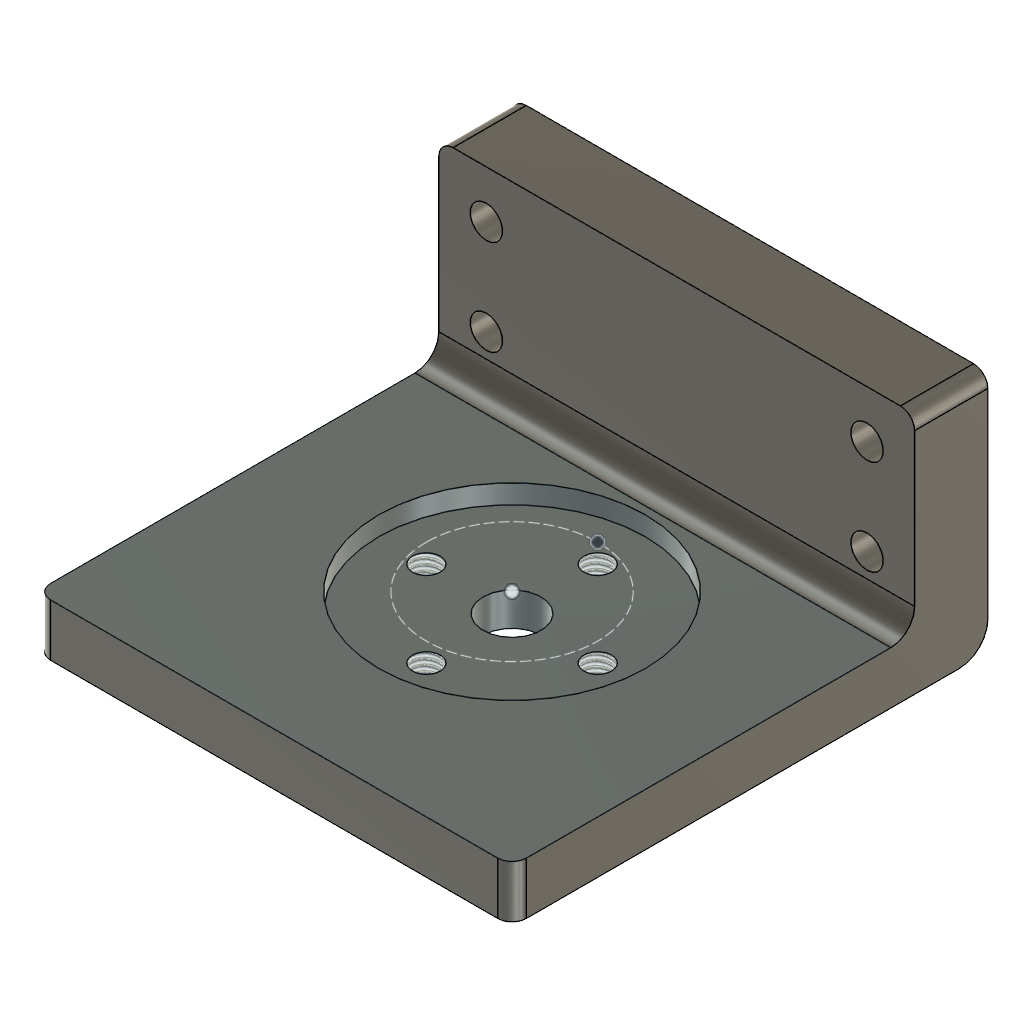
Motor Mount (Autodesk Fusion 360 design; units mm, degrees)
part number: 2026-09-16-15-06-11-104
Autodesk Fusion 360 part; units mm, degrees
sketch "Sketch1" plane through (0, 0, 0) normal (0, 0, 1) x (1, 0, 0)
  line L0 (25, 25) -> (-25, 25)
  line L1 (-25, 25) -> (-25, -25)
  line L2 (-25, -25) -> (25, -25)
  line L3 (25, -25) -> (25, 25)
  line L4 (25, 25) -> (-25, -25) construction
  line L5 (-25, 25) -> (25, -25) construction
  dimension "d1" = 50
  dimension "d2" = 50
  constraint horizontal L0
  constraint perpendicular L0 L1
  constraint parallel L0 L2
  constraint parallel L1 L3
  constraint coincident L4 origin
  constraint coincident L5 origin
  measures "d1" distance of L0.end L1.end
  measures "d2" distance of L0.start L0.end
extrude "Extrude1" add sketch "Sketch1" along normal blind 5.5
sketch "Sketch2" plane through (0, 0, 5.5) normal (0, 0, 1) x (-1, 0, 0)
  line L0 (-25, 25) -> (-25, -25)
  line L1 (-25, -25) -> (25, -25)
  line L2 (25, -25) -> (25, 25)
  line L3 (25, 25) -> (-25, 25)
  line L4 (25, -25) -> (-25, -25)
  line L5 (-25, -25) -> (-25, -17.3)
  line L6 (-25, -17.3) -> (25, -17.3)
  line L7 (25, -17.3) -> (25, -25)
  dimension "d11" = 7.7
  dimension "d12" = 50
  constraint horizontal L4
  constraint vertical L5
  constraint horizontal L6
  constraint vertical L7
  constraint coincident L1.end L2.start
  measures "d11" distance of L1.end L6.end
  measures "d12" distance of L1.end L0.end
extrude "Extrude2" add sketch "Sketch2" along normal blind 20 contours L0 L1 L2 L4 L5 L6 L7
sketch "Sketch3" plane through (0, 0, 5.5) normal (0, 0, 1) x (-1, 0, 0)
  line L0 (-25, -17.3) -> (25, -17.3)
  line L1 (25, -17.3) -> (25, 25)
  line L2 (25, 25) -> (-25, 25)
  line L3 (-25, 25) -> (-25, -17.3)
  circle A0 centre (0, 0) radius 14
  dimension "d15" = 28
  constraint coincident A0.centre origin
  measures "d15" diameter of A0
sketch "Sketch4" plane through (0, 0, 5.5) normal (0, 0, 1) x (-1, 0, 0)
fillet "Fillet1" radius 2.5 1 edges at (0, 17.3, 5.5)
fillet "Fillet2" radius 3 1 edges at (0, 25, 0)
fillet "Fillet3" radius 1.5 4 edges at (25, -25, 2.75) (-25, -25, 2.75) (25, 21.15, 25.5) (-25, 21.15, 25.5)
extrude "Extrude3" cut sketch "Sketch3" against normal blind 2 contours A0
sketch "Sketch5" plane through (0, 0, 5.5) normal (0, 0, 1) x (-1, 0, 0)
  circle A0 centre (0, 0) radius 14
  arc A1 (25, 23.5) -> (23.5, 25) centre (23.5, 23.5) ccw
  line L0 (23.5, 25) -> (-23.5, 25)
  arc A2 (-23.5, 25) -> (-25, 23.5) centre (-23.5, 23.5) ccw
  line L1 (-25, 23.5) -> (-25, -14.8)
  line L2 (-25, -14.8) -> (25, -14.8)
  line L3 (25, -14.8) -> (25, 23.5)
  circle A3 centre (0, 0) radius 9 construction
  point P0 (0, -9)
  dimension "d24" = 18
  constraint concentric A0 A3
  constraint coincident A3 P0
  measures "d24" diameter of A3
hole "Hole1" at (0, 0, 5.5) direction (0, 0, -1) diameter 6.1 depth 10 tip angle 118
hole "Hole2" at (0, 9, 5.5) direction (0, 0, -1) diameter 2.93 depth 10 tip angle 118
thread "Thread1" "ISO Metric profile 3.5 M3.5x0.6 M3.5x0.6 6H" thread offset 0 thread depth 7.4
pattern_circular "C-Pattern1" count 4 over 360 about axis through (0, 0, 1.75) along (0, 0, 1) of "Hole2"
hole "Hole3" at (-20, 17.3, 20.5) direction (0, 1, 0) diameter 3.4 depth 10 tip angle 118
hole "Hole4" at (-20, 17.3, 10.5) direction (0, 1, 0) diameter 3.4 depth 10 tip angle 118
hole "Hole5" at (20, 17.3, 20.5) direction (0, 1, 0) diameter 3.4 depth 10 tip angle 118
hole "Hole6" at (20, 17.3, 10.5) direction (0, 1, 0) diameter 3.4 depth 10 tip angle 118
equation "Base_Feature_1 = 50 mm"
equation "Width_Feature_1 = 50 mm"
equation "thickness_Feature_1 = 5.5 mm"
equation "Base_Feature_2 = 50 mm"
equation "Height_Feature_2 = 20 mm"
equation "Thickness_Feature_2 = 7.7 mm"
equation "d11 = Thickness_Feature_2"
equation "d12 = Base_Feature_2"
equation "d13 = Height_Feature_2"
equation "Feature_2_Edge = 5 mm"
equation "Feature_2_Top = 5.0 mm"
equation "Feat_2_Left_Holes_Xpos = Feature_2_Edge"
equation "Feat_2_Right_Holes_xpos = Base_Feature_2 - Feature_2_Edge"
equation "motor_hole = 6.1 mm"
equation "Feature_1_Hole_Count_Mount = 4"
equation "Feature_1_Motor_Hole = 6.1 mm"
equation "Feature_1_Motor_Mount_Hole_Size = 3 mm"
